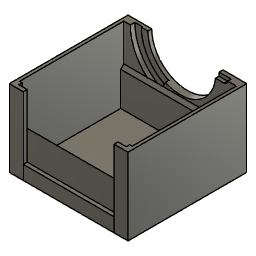
Deckbox - Lid (Autodesk Fusion 360 design; units mm, degrees)
Autodesk Fusion 360 part; units mm, degrees
sketch "Sketch1" plane through (0, 0, 0) normal (0, 1, 0) x (1, 0, 0)
  line L0 (2.25, 7.5) -> (82.75, 7.5)
  line L1 (82.75, 77.5) -> (2.25, 77.5)
  line L2 (2.25, 5.25) -> (82.75, 5.25)
  line L3 (82.75, 5.25) -> (82.75, 79.75)
  line L4 (82.75, 79.75) -> (2.25, 79.75)
  line L5 (2.25, 79.75) -> (2.25, 5.25)
  line L6 (4, 5.25) -> (81, 5.25)
  line L7 (81, 5.25) -> (81, 2.75)
  line L8 (81, 2.75) -> (4, 2.75)
  line L9 (4, 2.75) -> (4, 5.25)
  line L10 (4, 5.25) -> (0, 5.25)
  line L11 (0, 5.25) -> (0, 0)
  line L12 (0, 0) -> (10, 0)
  line L13 (10, 0) -> (10, 2.75)
  line L14 (81, 5.25) -> (85, 5.25)
  line L15 (85, 5.25) -> (85, 0)
  line L16 (85, 0) -> (75, 0)
  line L17 (75, 0) -> (75, 2.75)
  line L18 (0, 5.25) -> (85, 5.25)
  line L19 (85, 5.25) -> (85, 85)
  line L20 (85, 85) -> (0, 85)
  line L21 (0, 85) -> (0, 5.25)
  line L22 (10, 0) -> (75, 0)
  point P0 (42.5, 5.25)
  point P1 (42.5, 5.25)
  dimension "d5" = 2.25
  dimension "d7" = 2.25
  dimension "d19" = 77
  dimension "d27" = 10
  dimension "d29" = 5.25
  dimension "d30" = 2.25
  dimension "d58" = 5.25
  dimension "d59" = 2.5
  dimension "d61" = 10
  dimension "d62" = 2.25
  dimension "d76" = 85
  dimension "d77" = 85
  constraint horizontal L0
  constraint horizontal L1
  constraint horizontal L2
  constraint vertical L3
  constraint horizontal L4
  constraint vertical L5
  constraint horizontal L6
  constraint vertical L7
  constraint horizontal L8
  constraint vertical L9
  constraint perpendicular L9 L10
  constraint perpendicular L10 L11
  constraint perpendicular L11 L12
  constraint coincident L8 L13.end
  constraint perpendicular L8 L13
  constraint perpendicular L7 L14
  constraint perpendicular L14 L15
  constraint perpendicular L15 L16
  constraint coincident L8 L17.end
  constraint perpendicular L8 L17
  constraint midpoint L6 P1
  constraint midpoint L2 P1
  constraint coincident P1 P0
  constraint horizontal L18
  constraint vertical L19
  constraint horizontal L20
  constraint vertical L21
  constraint coincident L15 L14.end
  constraint horizontal L22
  constraint coincident L1.start L3
  constraint coincident L1.end L5
  constraint coincident L0.start L5
  constraint coincident L0.end L3
  constraint coincident L11.end L12.start
  measures "d5" distance of L1 L4
  measures "d7" distance of L0 L2
  measures "d19" distance of L6.start L6.end
  measures "d27" distance of L15 L17
  measures "d29" distance of L4 L20
  measures "d30" distance of L3 L19
  measures "d58" distance of L2 L22
  measures "d59" distance of L8 L18
  measures "d61" distance of L11 L13
  measures "d62" distance of L5 L21
  measures "d76" distance of L11.end L15.end
  measures "d77" distance of L11.end L20.end
extrude "Extrude1" add sketch "Sketch1" against normal blind 2
extrude "Extrude2" add sketch "Sketch1" along normal blind 26.5 contours L0 L2 L3 L5 L6 L10 L14 L18 | L1 L3 L4 L5
extrude "Extrude3" add sketch "Sketch1" along normal blind 53 contours L3 L4 L5 L10 L14 L18 L19 L20 L21 | L2 L8 L9 L10 L11 L12 L13 L18 | L2 L7 L8 L14 L15 L16 L17 L18
extrude "Extrude5" add sketch "Sketch1" along normal blind 8 contours L8 L13 L17 L22
extrude "Extrude10" add 1 faces at (55.3333, 0, -4.4167) along direction (0, 1, 0) blind 3
sketch "Sketch6" plane through (0, 0, -85) normal (0, 0, -1) x (-1, 0, 0)
  circle A0 centre (-42.5, 53) radius 25.5
  line L0 (0, 53) -> (-85, 53) construction
  point P0 (-42.5, 53)
  point P1 (0, 53)
  point P2 (-85, 53)
  dimension "d40" = 51
  constraint coincident P0 A0.centre
  constraint horizontal L0
  constraint midpoint P0 L0
  constraint coincident P1 L0.start
  constraint coincident P2 L0.end
  measures "d40" diameter of A0
extrude "Extrude7" cut sketch "Sketch6" against normal blind 5.25
sketch "Sketch7" plane through (0, 0, -85) normal (0, 0, -1) x (-1, 0, 0)
  circle A0 centre (-42.5, 53) radius 35.55
  circle A1 centre (-42.5, 53) radius 30.25
  circle A2 centre (-42.5, 53) radius 25.5
  line L0 (-26.4898, 25.2696) -> (-42.5, 53) construction
  circle A3 centre (-74.05, 53) radius 2.55
  line L1 (-74.05, 53) -> (-42.5, 53)
  line L2 (-42.5, 53) -> (-42.5, 50.45)
  line L3 (-42.5, 50.45) -> (-74.05, 50.45)
  line L4 (-74.05, 50.45) -> (-74.05, 53)
  line L5 (-44.6651, 51.75) -> (-42.5, 53)
  line L6 (-26.4898, 25.2696) -> (-28.6549, 24.0196)
  line L7 (-28.6549, 24.0196) -> (-44.6651, 51.75)
  circle A4 centre (-33.0344, 21.4911) radius 2.65
  circle A5 centre (-33.0551, 26.641) radius 2.5
  line L8 (-78.05, 53) -> (-74.05, 53)
  line L9 (-28.6549, 24.0196) -> (-33.0344, 21.4911)
  line L10 (-85, 53) -> (0, 53)
  point P0 (-85, 53)
  point P1 (0, 53)
  dimension "d52" = 51
  dimension "d55" = 5.1
  dimension "d67" = 5.3
  dimension "d71" = 5
  dimension "d72" = 4
  dimension "d81" = 2.5
  dimension "d82" = 60
  dimension "d85" = 60.5
  constraint horizontal L1
  constraint vertical L2
  constraint horizontal L3
  constraint vertical L4
  constraint coincident A3.centre L1.start
  constraint parallel L5 L6
  constraint tangent A0 A4
  constraint tangent A1 A4
  constraint tangent A4 A5
  constraint tangent L7 A5
  constraint tangent A2 A5
  constraint coincident A0 L8.start
  constraint tangent A3 L3
  constraint coincident A0.centre L2
  constraint coincident L0.start L6.start
  constraint perpendicular L0 L6
  constraint coincident A0.centre A1.centre
  constraint perpendicular L7 L9
  constraint coincident A4.centre L9.end
  constraint coincident P0 L10.start
  constraint coincident P1 L10.end
  constraint midpoint A0.centre L10
  constraint collinear L8 L10
  measures "d52" diameter of A2
  measures "d55" diameter of A3
  measures "d67" diameter of A4
  measures "d71" diameter of A5
  measures "d72" distance of A3.centre L8.start
  measures "d81" distance of L0 L7
  measures "d82" angle of L0 L10
  measures "d85" diameter of A1
extrude "Extrude8" cut sketch "Sketch7" along normal blind 3.2 from surface at -5.25 contours A0 A1 L7 A4 L9 L10 | A4 | A1 A4 A5 | A1 L7 A4 A5 L9 | A1 A5 picked at (-32.2182, 24.4659)
extrude "Extrude9" cut sketch "Sketch7" along normal blind 2.5 from surface at -5.25 contours A0 A1 L7 A4 L9 L10 | A1 A2 L7 L10 | A3 L4 L8 L10 | A1 A3 L1 L8 L10 | A1 A3 L1 L10 | A1 L7 A5 | A1 A3 L1 L4 L10 | A1 A3 L3 | A1 A2 A3 L1 L3 L10 | A1 A3 L1 L10 | A2 L1 L3 L5 L7 L10 | L2 L3 L5 L7
extrude "Extrude11" cut 1 faces at (55.3333, 3, -4.4167) along direction (0, -1, 0) blind 3
sketch "Sketch8" plane through (0, 26.5, 0) normal (0, 1, 0) x (-1, 0, 0)
  line L0 (-2.25, -79.75) -> (-2.25, -77.5)
  line L1 (-2.25, -5.25) -> (-4, -5.25)
  line L2 (-4, -5.25) -> (-81, -5.25)
  line L3 (-81, -5.25) -> (-82.75, -5.25)
  line L4 (-82.75, -77.5) -> (-82.75, -79.75)
  line L5 (-82.75, -79.75) -> (-30.5591, -79.75)
  line L6 (-30.5591, -79.75) -> (-18.8029, -79.75)
  line L7 (-4, -5.25) -> (-81, -5.25)
  line L8 (-81, -5.25) -> (-81, -5.5)
  line L9 (-81, -5.5) -> (-4, -5.5)
  line L10 (-4, -5.5) -> (-4, -5.25)
  line L11 (-18.8029, -79.75) -> (-2.25, -79.75)
  line L12 (-2.25, -77.5) -> (-82.75, -77.5)
  line L13 (-2.25, -7.5) -> (-2.25, -5.25)
  line L14 (-82.75, -5.25) -> (-82.75, -7.5)
  line L15 (-82.75, -7.5) -> (-2.25, -7.5)
  dimension "d78" = 0.25
  constraint horizontal L7
  constraint vertical L8
  constraint horizontal L9
  constraint vertical L10
  constraint coincident L1.end L2.start
  constraint coincident L2.end L8
  measures "d78" distance of L7 L9
extrude "Extrude12" cut sketch "Sketch8" against normal blind 26 contours L2 L7 L8 L9 L10
chamfer "Chamfer2" distance 2.25 angle 45 2 edges at (42.5, 26.5, -77.5) (42.5, 26.5, -7.5)
equation "d69 = 0 mm - 5.25 mm"
named bodies: "Deckbox - Lid"
